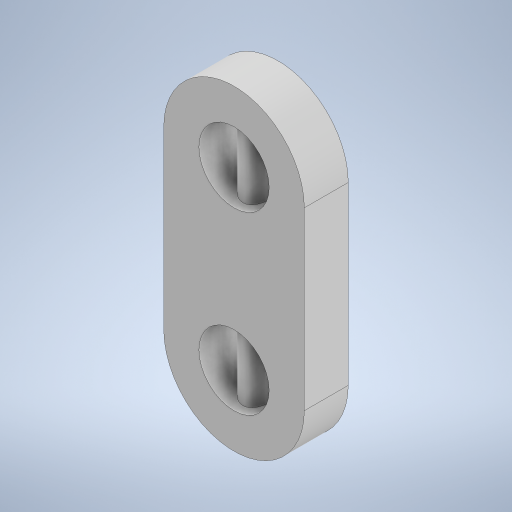
# Autodesk Inventor part: 1-16
Saved by Autodesk Inventor 2024.2 (Build 282272000, 272)
## iProperties
Created: 2024-10-10
Part Number: 1-16
Material: Generic
Document SubType Name: Modeling
Designer: Precisión-04
Density: 1 g/cm^3
Appearance: Default
Author: Precisión-04
Autodesk Inventor part; units mm, degrees
ref_plane "YZ Plane" through (0, 0, 0) normal (1, 0, 0) x (0, 1, 0)
ref_plane "XZ Plane" through (0, 0, 0) normal (0, 1, 0) x (-1, 0, 0)
ref_plane "XY Plane" through (0, 0, 0) normal (0, 0, 1) x (1, 0, 0)
sketch "Sketch1" plane through (0, 0, 0) normal (0, 0, 1) x (1, 0, 0)
  arc A0 (4, 0) -> (-4, 0) centre (0, 0) ccw
  line L0 (0, 0) -> (0, -10) construction
  line L1 (-4, 0) -> (-4, -10)
  line L2 (4, 0) -> (4, -10)
  arc A1 (-4, -10) -> (4, -10) centre (0, -10) ccw
  circle A2 centre (0, 0) radius 2
  circle A3 centre (0, -10) radius 2
  dimension "d0" = 8
  dimension "d2" = 8
  dimension "d3" = 10
  dimension "d4" = 4
  dimension "d5" = 4
  constraints: 6 end point, 4 centre point, 4 coincident, 4 point on circle, 3 vertical, 2 tangent
  measures "d0" diameter of A0
  measures "d2" diameter of A1
  measures "d3" distance of point (0, 0) L0.end
  measures "d4" diameter of A2
  measures "d5" diameter of A3
extrude "Extrusion1" add sketch "Sketch1" along normal blind 2.5
sketch "Sketch4" plane through (0, 0, 0) normal (1, 0, 0) x (0, 1, 0)
  line L0 (2, 2.5) -> (2, 0) projected
  line L1 (-2, 2.5) -> (-2, 0) projected
  line L2 (2, 1.25) -> (-2, 1.25)
  line L3 (-2, 1.25) -> (-2, 2)
  line L4 (-2, 2) -> (2, 2)
  line L5 (2, 2) -> (2, 1.25)
  point P0 (0, 0)
  dimension "d14" = 1.5
  constraints: 8 end point, 2 parallel, 1 horizontal, 1 midpoint, 1 perpendicular, 1 point on line
  measures "d14" diameter of L4 L2
revolve "Revolution1" add sketch "Sketch4" angle 360 about axis through (0, 2, 1.25) along (0, -1, 0)
sketch "Sketch5" plane through (0, 0, 0) normal (1, 0, 0) x (0, 1, 0)
  line L0 (-8, 2.5) -> (-8, 0) projected
  line L1 (-12, 2.5) -> (-12, 0) projected
  line L2 (-8, 1.25) -> (-12, 1.25)
  line L3 (-12, 1.25) -> (-12, 2)
  line L4 (-12, 2) -> (-8, 2)
  line L5 (-8, 2) -> (-8, 1.25)
  point P0 (0, 0)
  dimension "d16" = 1.5
  constraints: 8 end point, 2 parallel, 1 horizontal, 1 midpoint, 1 perpendicular, 1 point on line
  measures "d16" diameter of L4 L2
revolve "Revolution2" add sketch "Sketch5" angle 360 about axis through (0, -8, 1.25) along (0, -1, 0)
body "Solid1"
